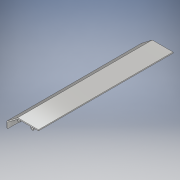
# Autodesk Inventor part: DriveBaseFront
Saved by Autodesk Inventor 2017 (Build 210142000, 142)
## iProperties
Created: 2017-04-25
Part Number: DriveBaseFront
Material: Generic
Document SubType Name: Modeling
Designer: admin
Density: 1 g/cm^3
Appearance: Aluminum - Polished
Author: admin
Autodesk Inventor part; units mm, degrees
ref_plane "YZ Plane" through (0, 0, 0) normal (1, 0, 0) x (0, 1, 0)
ref_plane "XZ Plane" through (0, 0, 0) normal (0, 1, 0) x (-1, 0, 0)
ref_plane "XY Plane" through (0, 0, 0) normal (0, 0, 1) x (1, 0, 0)
ref_plane "Work Plane1" through (0, -383.0536, 0) normal (0, 0, 1) x (1, 0, 0)
sketch "Sketch1" plane through (0, -383.0536, 0) normal (0, 0, 1) x (1, 0, 0)
  line L0 (41.7899, 534.0845) -> (106.8774, 534.0845) projected
  line L1 (14.8024, 513.5226) -> (41.7899, 534.0845) projected
  line L2 (106.8774, 530.9095) -> (42.8616, 530.9095)
  line L3 (42.8616, 530.9095) -> (16.7266, 510.9971)
  line L4 (106.8774, 534.0845) -> (106.8774, 530.9095)
  line L5 (11.6274, 489.6345) -> (11.6274, 207.8533) projected
  line L6 (16.7266, 510.9971) -> (11.6274, 507.112)
  line L7 (14.8024, 513.5226) -> (8.4524, 508.6845)
  line L8 (11.6274, 489.6345) -> (11.6274, 507.112)
  line L9 (11.6274, 489.6345) -> (11.6274, 207.8533) projected
  line L10 (8.4524, 489.6345) -> (8.4524, 207.8533) projected
  line L11 (11.6274, 489.6345) -> (8.4524, 489.6345) projected
  line L12 (8.4524, 489.6345) -> (8.4524, 508.6845)
  point P0 (0, 383.0536)
  dimension "d0" = 3.175
  constraints: 14 end point, 3 vertical, 1 collinear, 1 other
  measures "d0" distance between parallel lines of L0 L2
extrude "Extrusion1" add sketch "Sketch1" along normal blind 420.497
sketch "Sketch2" plane through (0, -383.0536, 420.497) normal (0, 0, 1) x (1, 0, 0)
  line L0 (42.8616, 530.9095) -> (106.8774, 530.9095) projected
  line L1 (92.9074, 530.9095) -> (82.7474, 530.9095)
  arc A0 (82.7474, 528.3695) -> (92.9074, 528.3695) centre (87.8274, 528.3695) ccw
  line L2 (106.8774, 534.0845) -> (41.7899, 534.0845) projected
  arc A1 (89.5122, 530.9095) -> (86.1425, 530.9095) centre (87.8274, 528.3695) ccw
  line L3 (92.9074, 528.3695) -> (92.9074, 530.9095)
  line L4 (82.7474, 530.9095) -> (82.7474, 528.3695)
  arc A2 (83.428, 530.9095) -> (82.7474, 528.3695) centre (87.8274, 528.3695) ccw construction
  arc A3 (92.2268, 530.9095) -> (83.428, 530.9095) centre (87.8274, 528.3695) ccw
  arc A4 (92.9074, 528.3695) -> (92.2268, 530.9095) centre (87.8274, 528.3695) ccw construction
  arc A5 (86.1425, 530.9095) -> (89.5122, 530.9095) centre (87.8274, 528.3695) ccw
  line L5 (41.1835, 533.6226) -> (43.2506, 530.9095)
  line L6 (14.8024, 513.5226) -> (41.7899, 534.0845) projected
  arc A6 (40.1058, 528.3695) -> (50.2658, 528.3695) centre (45.1858, 528.3695) ccw
  arc A7 (43.501, 530.9095) -> (46.8707, 530.9095) centre (45.1858, 528.3695) ccw
  line L7 (50.2658, 528.3695) -> (50.2658, 530.9095)
  line L8 (11.6274, 507.112) -> (42.8616, 530.9095) projected
  line L9 (40.1058, 528.3695) -> (40.1058, 528.8099)
  line L10 (43.2506, 530.9095) -> (43.3386, 530.794) construction
  arc A8 (40.1264, 528.8256) -> (40.1058, 528.3695) centre (45.1858, 528.3695) ccw construction
  arc A9 (49.5853, 530.9095) -> (40.1264, 528.8256) centre (45.1858, 528.3695) ccw
  arc A10 (50.2658, 528.3695) -> (49.5853, 530.9095) centre (45.1858, 528.3695) ccw construction
  arc A11 (46.8707, 530.9095) -> (43.501, 530.9095) centre (45.1858, 528.3695) ccw
  point P0 (0, 383.0536)
  dimension "d3" = 10.16
  dimension "d4" = 13.97
  dimension "d5" = 10.16
  dimension "d8" = 6.096
  dimension "d9" = 5.715
  dimension "d10" = 3.556
  dimension "d11" = 10.16
  dimension "d12" = 6.096
  dimension "d13" = 5.715
  constraints: 27 point on circle, 14 end point, 12 centre point, 12 tangent, 7 point on line, 3 vertical, 2 coincident, 2 line through centre, 2 perpendicular, 8 other
  measures "d3" distance of L1.start L1.end
  measures "d4" distance of L1.start point (106.877, 530.91)
  measures "d5" diameter of A0
  measures "d8" diameter of A1
  measures "d9" distance from line of L2 A1.centre
  measures "d10" distance of L5.start L10.end
  measures "d11" diameter of A6
  measures "d12" diameter of A7
  measures "d13" distance from line of L2 A6.centre
extrude "Extrusion2" add sketch "Sketch2" against normal up to surface (420.497 mm away) contours L0 A7 L7 A6 L9 L8 | L0 A5 L3 A0 L4
body "Solid1"
